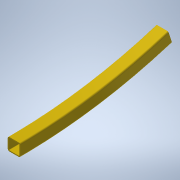
# Autodesk Inventor part: Lacznik zaokraglony
Saved by Autodesk Inventor 2021 (Build 250183000, 183)
## iProperties
Created: 2024-04-08
Part Number: Lacznik zaokraglony
Material: Steel
Document SubType Name: Modeling
Designer: Michal
Density: 7.85 g/cm^3
Appearance: Glossy - Gold
Author: Michal
Autodesk Inventor part; units mm, degrees
ref_plane "YZ Plane" through (0, 0, 0) normal (1, 0, 0) x (0, 1, 0)
ref_plane "XZ Plane" through (0, 0, 0) normal (0, 1, 0) x (-1, 0, 0)
sketch "Sketch1" plane through (0, 0, 0) normal (0, 1, 0) x (-1, 0, 0)
  line L0 (-9.5, 11.5) -> (9.5, 11.5) construction
  line L1 (11.5, 9.5) -> (11.5, -9.5) construction
  line L2 (9.5, -11.5) -> (-9.5, -11.5) construction
  line L3 (-11.5, -9.5) -> (-11.5, 9.5) construction
  line L4 (-11.5, 11.5) -> (11.5, -11.5) construction
  line L5 (11.5, 11.5) -> (-11.5, -11.5) construction
  arc A0 (11.5, 9.5) -> (9.5, 11.5) centre (9.5, 9.5) ccw construction
  arc A1 (9.5, -11.5) -> (11.5, -9.5) centre (9.5, -9.5) ccw construction
  arc A2 (-11.5, -9.5) -> (-9.5, -11.5) centre (-9.5, -9.5) ccw construction
  arc A3 (-9.5, 11.5) -> (-11.5, 9.5) centre (-9.5, 9.5) ccw construction
  line L6 (-9.5, -12.5) -> (9.5, -12.5)
  arc A4 (9.5, -12.5) -> (12.5, -9.5) centre (9.5, -9.5) ccw
  line L7 (12.5, -9.5) -> (12.5, 9.5)
  arc A5 (12.5, 9.5) -> (9.5, 12.5) centre (9.5, 9.5) ccw
  line L8 (9.5, 12.5) -> (-9.5, 12.5)
  arc A6 (-9.5, 12.5) -> (-12.5, 9.5) centre (-9.5, 9.5) ccw
  line L9 (-12.5, 9.5) -> (-12.5, -9.5)
  arc A7 (-12.5, -9.5) -> (-9.5, -12.5) centre (-9.5, -9.5) ccw
  line L10 (10.5, -9.5) -> (10.5, 9.5)
  arc A8 (10.5, 9.5) -> (9.5, 10.5) centre (9.5, 9.5) ccw
  line L11 (9.5, 10.5) -> (-9.5, 10.5)
  arc A9 (-9.5, 10.5) -> (-10.5, 9.5) centre (-9.5, 9.5) ccw
  line L12 (-10.5, 9.5) -> (-10.5, -9.5)
  arc A10 (-10.5, -9.5) -> (-9.5, -10.5) centre (-9.5, -9.5) ccw
  line L13 (-9.5, -10.5) -> (9.5, -10.5)
  arc A11 (9.5, -10.5) -> (10.5, -9.5) centre (9.5, -9.5) ccw
  point P0 (0, 0)
  point P1 (0, 0)
  point P2 (0, 0)
  dimension "d10" = 2
  dimension "depth" = 25
  dimension "width" = 25
  dimension "thickness" = 2
  constraints: 28 end point, 24 point on circle, 12 centre point, 8 point on line, 8 tangent, 6 parallel, 3 equal radius, 3 midpoint, 3 perpendicular, 1 coincident, 1 horizontal, 15 other
  measures "d10" radius of A0
  measures "depth" distance between parallel lines of L6 L8
  measures "width" distance between parallel lines of L9 L7
  measures "thickness" distance between parallel lines of L10 L7
sketch "Sketch3" plane through (0, 0, 0) normal (1, 0, 0) x (0, 1, 0)
  line L0 (0, 0) -> (0, 2000) construction
  arc A0 (0, 0) -> (300, 46.0608) centre (0, 1000) ccw
  line L1 (0, -413.7378) -> (0, 2402.2896) projected
  line L2 (-62.8971, 0) -> (377.3825, 0) projected
  line L3 (0, 1000) -> (314.4855, 0) construction
  dimension "d30" = 2000
  dimension "d31" = 1000
  dimension "d61" = 300
  constraints: 4 end point, 4 point on line, 2 point on circle, 1 centre point, 1 collinear
  measures "d30" distance of L0.start L0.end
  measures "d31" radius of A0
  measures "d61" distance from line of L3 point (0, 0)
sweep "Sweep1" add profiles "Sketch1" path "Sketch3" path curves A0
ref_plane "Work Plane3" through (-9.5, 0, 1000) normal (0, -0.9884, -0.1518) x (1, 0, 0)
sketch "Sketch5" plane through (-12.5, 0, 1000) normal (-1, 0, 0) x (0, 0.9884, 0.1518)
  arc A0 (151.7577, -988.4177) -> (-151.7577, 988.4177) centre (0, 0) ccw construction
  line L0 (-153.1994, 997.8077) -> (-150.316, 979.0278) projected
  line L1 (153.1994, 997.8077) -> (150.316, 979.0278) projected
  line L2 (0, -1863.5732) -> (0, 2015.3309) construction
  point P0 (-1000, 0)
  point P1 (-99.8594, 995.0016)
  point P2 (-50, 998.7492)
  point P3 (1000, 0)
  point P4 (99.8594, 995.0016)
  point P5 (50, 998.7492)
  point P6 (150.316, 979.0278)
  dimension "d51" = 50
  dimension "d53" = 50
  dimension "d62" = 100
  constraints: 1 symmetric about line, 9 other
  measures "d51" distance of point (99.859, 995.002) point (50, 998.749)
  measures "d53" distance of point (-50, 998.749) point (-99.859, 995.002)
  measures "d62" distance of point (-50, 998.749) point (50, 998.749)
hole "Hole3" at (-12.5, 52.2964, 1.3684) at (-12.5, 102.147, 5.2307) at (-12.5, 249.7019, 31.6772) at (-12.5, 200.9888, 20.4065) direction (1, 0, 0) diameter 6.647 depth 22.2 tip angle 118
equation "\"d10\" = thickness"
equation "\"d31\" = 0.5 * d30"
body "Solid2"
